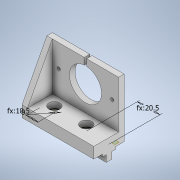
# Autodesk Inventor part: Pump_Mount
Saved by Autodesk Inventor 2022 (Build 260153000, 153)
## iProperties
Created: 2024-03-14
Part Number: Pump_Mount
Material: Generic
Document SubType Name: Modeling
Designer: Gotham City
Density: 1 g/cm^3
Appearance: Default
Author: Gotham City
Autodesk Inventor part; units mm, degrees
ref_plane "YZ Plane" through (0, 0, 0) normal (1, 0, 0) x (0, 1, 0)
ref_plane "XZ Plane" through (0, 0, 0) normal (0, 1, 0) x (-1, 0, 0)
ref_plane "XY Plane" through (0, 0, 0) normal (0, 0, 1) x (1, 0, 0)
sketch "Sketch1" plane through (0, 0, 0) normal (0, 0, 1) x (1, 0, 0)
  line L0 (-60, 0) -> (0, 0)
  line L1 (0, 0) -> (0, 10)
  line L2 (0, 10) -> (-60, 10)
  line L3 (-60, 10) -> (-60, 0)
  dimension "d1" = 10
  dimension "d59" = 60
  constraints: 8 end point, 2 horizontal, 1 perpendicular, 1 vertical
  measures "d1" distance of L0.end L1.end
  measures "d59" distance of L1.end L2.end
extrude "Extrusion1" add sketch "Sketch1" along normal mid plane 27.5
sketch "Sketch2" plane through (-60, 0, 13.75) normal (0, -1, 0) x (1, 0, 0)
  line L0 (0, -27.5) -> (0, 0) projected
  line L1 (60, 0) -> (60, -27.5) projected
  line L2 (0, -7.75) -> (60, -7.75)
  line L3 (60, -7.75) -> (60, -19.75)
  line L4 (60, -19.75) -> (0, -19.75)
  line L5 (0, -19.75) -> (0, -7.75)
  line L6 (30, -7.75) -> (30, 0) construction
  line L7 (0, 0) -> (60, 0) construction
  line L8 (0, -27.5) -> (60, -27.5) construction
  line L9 (30, -27.5) -> (30, -19.75) construction
  point P0 (60, -13.75)
  point P1 (0, -19.75)
  dimension "d4" = 12
  constraints: 14 end point, 4 midpoint, 2 parallel, 2 point on line, 1 collinear, 1 horizontal, 1 perpendicular
  measures "d4" distance between parallel lines of L4 L2
extrude "Extrusion2" add sketch "Sketch2" along normal blind 2.2
sketch "Sketch3" plane through (-60, -2.2, 13.75) normal (0, -1, 0) x (1, 0, 0)
  line L0 (0, -7.75) -> (0, -19.75) projected
  line L1 (60, -27.5) -> (60, 0) projected
  line L2 (0, -11.25) -> (60, -11.25)
  line L3 (60, -11.25) -> (60, -16.25)
  line L4 (60, -16.25) -> (0, -16.25)
  line L5 (0, -16.25) -> (0, -11.25)
  line L6 (30, -11.25) -> (30, -7.75) construction
  line L7 (0, -19.75) -> (60, -19.75) construction
  line L8 (30, -19.75) -> (30, -16.25) construction
  line L9 (60, -7.75) -> (0, -7.75) construction
  point P0 (60, -13.75)
  point P1 (0, -16.25)
  dimension "d7" = 5
  constraints: 12 end point, 4 midpoint, 2 parallel, 2 point on line, 1 collinear, 1 horizontal, 1 perpendicular, 1 vertical
  measures "d7" distance between parallel lines of L4 L2
extrude "Extrusion3" add sketch "Sketch3" along normal blind 6
ref_plane "Work Plane2" through (-60, 4.8, 13.75) normal (0, -1, 0) x (1, 0, 0)
sketch "Sketch4" plane through (-60, 4.8, 13.75) normal (0, -1, 0) x (1, 0, 0)
  circle A0 centre (10.5, -13.75) radius 4.5
  circle A1 centre (39.5, -13.75) radius 4.5
  line L0 (10.5, -13.75) -> (0, -13.75) construction
  line L1 (60, -16.25) -> (0, -16.25) construction
  line L2 (39.5, -13.75) -> (10.5, -13.75) construction
  line L3 (60, -11.25) -> (0, -11.25) construction
  line L4 (39.5, -13.75) -> (60, -13.75) construction
  line L5 (0, -11.25) -> (0, -16.25) construction
  dimension "d12" = 9
  dimension "d14" = 10.5
  dimension "d30" = 20.5
  constraints: 6 end point, 2 centre point, 2 parallel, 1 equal radius, 1 horizontal, 1 midpoint
  measures "d12" diameter of A0
  measures "d14" distance from line of L5 L0.start
  measures "d30" distance of L2.start L4.end
hole "Hole1" at (-49.5, 4.8, 0) at (-20.5, 4.8, 0) direction (0, -1, 0) diameter 5.5 end through all start extended yes counterbore diameter 10 counterbore depth 0.1 clearance for "Socket Head Cap Screw ISO 4762" size "M5" standard "ISO"
sketch "Sketch5" plane through (-21.6456, -2.2, -2.5) normal (0, 0, -1) x (-1, 0, 0)
  line L0 (38.3544, 0) -> (-21.6456, 0) projected
  line L1 (23.3544, 0) -> (33.3544, 0)
  line L2 (33.3544, 0) -> (33.3544, -6)
  line L3 (33.3544, -6) -> (23.3544, -6)
  line L4 (23.3544, -6) -> (23.3544, 0)
  line L5 (3.3544, 0) -> (-5.6456, 0)
  line L6 (-5.6456, 0) -> (-5.6456, -6)
  line L7 (-5.6456, -6) -> (3.3544, -6)
  line L8 (3.3544, -6) -> (3.3544, 0)
  line L9 (0, -6) -> (26.7087, -6) construction
  line L10 (-21.6456, 7) -> (38.3544, 7) construction
  line L11 (23.3544, 7) -> (32.3544, 7) projected
  point P0 (33.3544, 7)
  point P1 (42.3544, 7)
  point P2 (-5.6456, 7)
  point P3 (3.3544, 7)
  constraints: 16 end point, 4 parallel, 4 vertical alignment, 3 point on line, 2 horizontal, 2 perpendicular, 1 horizontal alignment
extrude "Extrusion5" cut sketch "Sketch5" along normal through all both and the other way through all
sketch "Sketch7" plane through (-25, -2.2, -2.5) normal (0, 0, -1) x (-1, 0, 0)
  line L0 (35, -6) -> (30, -6) projected
  line L1 (30, 0) -> (30, -6) projected
  line L2 (35, -6) -> (30, -6)
  line L3 (30, -6) -> (30, 0)
  line L4 (30, 0) -> (35, 0)
  line L5 (35, 0) -> (35, -6)
  line L6 (35, 0) -> (-25, 0) projected
  line L7 (20, 0) -> (14, -6)
  line L8 (20, -6) -> (0, -6) projected
  line L9 (20, -6) -> (20, 0) projected
  line L10 (14, -6) -> (20, -6)
  line L11 (20, -6) -> (20, 0)
  line L12 (-9, 0) -> (-9, -6) projected
  line L13 (-9, -6.0008) -> (-9, 0)
  line L14 (-9, 0) -> (-15, -6)
  line L15 (-25, -6) -> (-9, -6) projected
  line L16 (-15, -6) -> (-9, -6)
  point P0 (-25, 2.2)
  dimension "d40" = 45
  dimension "d41" = 45
  constraints: 20 end point, 4 point on line, 3 horizontal, 2 parallel, 2 perpendicular, 1 collinear
  measures "d40" angle of L9 L7
  measures "d41" angle of L14 L13
extrude "Extrusion7" cut sketch "Sketch7" against normal through all
sketch "Sketch9" plane through (0, 0, -13.75) normal (0, 0, -1) x (-1, 0, 0)
  line L0 (0, 0) -> (0, 10) projected
  line L1 (0, 0) -> (60, 0)
  line L2 (60, 0) -> (60, 53)
  line L3 (60, 53) -> (0, 53)
  line L4 (0, 53) -> (0, 0)
  circle A0 centre (30, 32.5) radius 14.5
  circle A1 centre (5.75, 32.5) radius 1.5
  line L5 (30, 32.5) -> (5.75, 32.5) construction
  line L6 (30, 18) -> (30, 47) construction
  circle A2 centre (54.25, 32.5) radius 1.5
  line L7 (0, 18) -> (60, 18) construction
  line L8 (60, 10) -> (0, 10) construction
  line L9 (0, 47) -> (60, 47) construction
  point P0 (60, 0)
  dimension "d60" = 29
  dimension "d61" = 3
  dimension "d68" = 48.5
  dimension "d70" = 8
  dimension "d71" = 6
  constraints: 16 end point, 3 centre point, 3 point on line, 3 symmetric about line, 2 horizontal, 2 midpoint, 2 parallel, 2 perpendicular, 2 point on circle, 1 coincident, 1 tangent, 1 vertical, 1 other
  measures "d60" diameter of A0
  measures "d61" diameter of A1
  measures "d68" distance of L5.end A2.centre
  measures "d70" distance between parallel lines of L7 L8
  measures "d71" distance between parallel lines of L3 L9
extrude "Extrusion9" add sketch "Sketch9" against normal blind 5
sketch "Sketch10" plane through (-60, 0, 13.75) normal (-1, 0, 0) x (0, 0, 1)
  line L0 (-27.5, 0) -> (-19.75, 0) projected
  line L1 (-19.75, 0) -> (-19.75, -2.2) projected
  line L2 (-7.75, -2.2) -> (-19.75, -2.2) projected
  line L3 (-7.75, 0) -> (-7.75, -2.2) projected
  line L4 (-7.75, 0) -> (0, 0) projected
  line L5 (0, 10) -> (0, 0) projected
  line L6 (-22.5, 10) -> (0, 10) construction
  line L7 (-22.5, 53) -> (-22.5, 10) construction
  line L8 (-27.5, 53) -> (-22.5, 53) projected
  line L9 (-27.5, 0) -> (-27.5, 53) projected
  line L10 (-22.5, 53) -> (-22.5, 10) construction
  line L11 (0, 0) -> (0, 10) construction
  line L12 (-22.5, 53) -> (0, 10)
  constraints: 2 end point
extrude "Extrusion10" add sketch "Sketch10" along normal blind 5
sketch "Sketch12" plane through (0, 0, -13.75) normal (0, 0, -1) x (-1, 0, 0)
  circle A0 centre (30, 32.5) radius 14.5 construction
  line L0 (30, 32.5) -> (30, 52.9913) construction
  line L1 (29, 32.5) -> (31, 32.5)
  line L2 (31, 32.5) -> (31, 53)
  line L3 (31, 53) -> (29, 53)
  line L4 (29, 53) -> (29, 32.5)
  line L5 (65, 53) -> (0, 53) projected
  point P0 (0, 0)
  dimension "d74" = 2
  constraints: 10 end point, 2 parallel, 1 horizontal, 1 midpoint, 1 perpendicular, 1 point on line, 1 vertical
  measures "d74" distance between parallel lines of L2 L4
extrude "Extrusion11" cut sketch "Sketch12" against normal through all
equation "\"d41\" = d40"
body "Solid1"
